j12 (Autodesk Fusion 360 design; units mm, degrees)
part number: 2026-05-31-16-27-39-001
Autodesk Fusion 360 part; units mm, degrees
sketch "Sketch1" plane through (0, 0, 0) normal (0, 0, 1) x (1, 0, 0)
  line L0 (0, 0) -> (50, 0)
  line L1 (50, 0) -> (50, 110)
  line L2 (50, 110) -> (0, 110)
  line L3 (0, 110) -> (0, 0)
  dimension "d1" = 50
  dimension "d2" = 110
  constraint horizontal L0
  constraint vertical L1
  constraint horizontal L2
  constraint vertical L3
  constraint coincident L0.start L3.end
  measures "d1" distance of L0.start L0.end
  measures "d2" distance of L0.start L2.end
extrude "Extrude1" add sketch "Sketch1" along normal blind 5
sketch "Sketch2" plane through (0, 0, 5) normal (0, 0, 1) x (-1, 0, 0)
  line L0 (0, -110) -> (0, 0)
  line L1 (0, 0) -> (-50, 0)
  line L2 (-50, 0) -> (-50, -110)
  line L3 (-50, -110) -> (0, -110)
  circle A0 centre (-5, -5) radius 4
  circle A1 centre (-15, -5) radius 4
  circle A2 centre (-25, -5) radius 4
  circle A3 centre (-35, -5) radius 4
  circle A4 centre (-45, -5) radius 4
  circle A5 centre (-5, -15) radius 4
  circle A6 centre (-15, -15) radius 4
  circle A7 centre (-25, -15) radius 4
  circle A8 centre (-35, -15) radius 4
  circle A9 centre (-45, -15) radius 4
  circle A10 centre (-25, -35) radius 4
  circle A11 centre (-5, -25) radius 4
  circle A12 centre (-35, -35) radius 4
  circle A13 centre (-5, -35) radius 4
  circle A14 centre (-25, -25) radius 4
  circle A15 centre (-15, -25) radius 4
  circle A16 centre (-45, -25) radius 4
  circle A17 centre (-35, -25) radius 4
  circle A18 centre (-45, -35) radius 4
  circle A19 centre (-15, -35) radius 4
  circle A20 centre (-5, -75) radius 4
  circle A21 centre (-25, -65) radius 4
  circle A22 centre (-45, -65) radius 4
  circle A23 centre (-45, -75) radius 4
  circle A24 centre (-5, -65) radius 4
  circle A25 centre (-35, -75) radius 4
  circle A26 centre (-35, -65) radius 4
  circle A27 centre (-25, -75) radius 4
  circle A28 centre (-15, -75) radius 4
  circle A29 centre (-35, -55) radius 4
  circle A30 centre (-15, -65) radius 4
  circle A31 centre (-15, -45) radius 4
  circle A32 centre (-5, -45) radius 4
  circle A33 centre (-25, -55) radius 4
  circle A34 centre (-15, -55) radius 4
  circle A35 centre (-25, -45) radius 4
  circle A36 centre (-45, -45) radius 4
  circle A37 centre (-5, -55) radius 4
  circle A38 centre (-45, -55) radius 4
  circle A39 centre (-35, -45) radius 4
  circle A40 centre (-15, -105) radius 4
  circle A41 centre (-5, -95) radius 4
  circle A42 centre (-45, -105) radius 4
  circle A43 centre (-45, -95) radius 4
  circle A44 centre (-25, -105) radius 4
  circle A45 centre (-15, -95) radius 4
  circle A46 centre (-45, -85) radius 4
  circle A47 centre (-25, -85) radius 4
  circle A48 centre (-35, -85) radius 4
  circle A49 centre (-35, -105) radius 4
  circle A50 centre (-35, -95) radius 4
  circle A51 centre (-25, -95) radius 4
  circle A52 centre (-5, -105) radius 4
  circle A53 centre (-5, -85) radius 4
  circle A54 centre (-15, -85) radius 4
  dimension "d5" = 8
  dimension "d6" = 8
  dimension "d7" = 8
  dimension "d8" = 8
  dimension "d9" = 8
  dimension "d10" = 8
  dimension "d11" = 8
  dimension "d12" = 8
  dimension "d13" = 8
  dimension "d14" = 8
  dimension "d15" = 8
  dimension "d16" = 8
  dimension "d17" = 8
  dimension "d18" = 8
  dimension "d19" = 8
  dimension "d20" = 8
  dimension "d21" = 8
  dimension "d22" = 8
  dimension "d23" = 8
  dimension "d24" = 8
  dimension "d25" = 8
  dimension "d26" = 8
  dimension "d27" = 8
  dimension "d28" = 8
  dimension "d29" = 8
  dimension "d30" = 8
  dimension "d31" = 8
  dimension "d32" = 8
  dimension "d33" = 8
  dimension "d34" = 8
  dimension "d35" = 8
  dimension "d36" = 8
  dimension "d37" = 8
  dimension "d38" = 8
  dimension "d39" = 8
  dimension "d40" = 8
  dimension "d41" = 8
  dimension "d42" = 8
  dimension "d43" = 8
  dimension "d44" = 8
  dimension "d45" = 8
  dimension "d46" = 8
  dimension "d47" = 8
  dimension "d48" = 8
  dimension "d49" = 8
  dimension "d50" = 8
  dimension "d51" = 8
  dimension "d52" = 8
  dimension "d53" = 8
  dimension "d54" = 8
  dimension "d55" = 8
  dimension "d56" = 8
  dimension "d57" = 8
  dimension "d58" = 8
  dimension "d59" = 8
  measures "d5" diameter of A0
  measures "d6" diameter of A1
  measures "d7" diameter of A2
  measures "d8" diameter of A3
  measures "d9" diameter of A4
  measures "d10" diameter of A5
  measures "d11" diameter of A6
  measures "d12" diameter of A7
  measures "d13" diameter of A8
  measures "d14" diameter of A9
  measures "d15" diameter of A11
  measures "d16" diameter of A15
  measures "d17" diameter of A14
  measures "d18" diameter of A17
  measures "d19" diameter of A16
  measures "d20" diameter of A13
  measures "d21" diameter of A19
  measures "d22" diameter of A10
  measures "d23" diameter of A12
  measures "d24" diameter of A18
  measures "d25" diameter of A32
  measures "d26" diameter of A31
  measures "d27" diameter of A35
  measures "d28" diameter of A39
  measures "d29" diameter of A36
  measures "d30" diameter of A37
  measures "d31" diameter of A34
  measures "d32" diameter of A33
  measures "d33" diameter of A29
  measures "d34" diameter of A38
  measures "d35" diameter of A24
  measures "d36" diameter of A30
  measures "d37" diameter of A21
  measures "d38" diameter of A26
  measures "d39" diameter of A22
  measures "d40" diameter of A20
  measures "d41" diameter of A28
  measures "d42" diameter of A27
  measures "d43" diameter of A25
  measures "d44" diameter of A23
  measures "d45" diameter of A53
  measures "d46" diameter of A54
  measures "d47" diameter of A47
  measures "d48" diameter of A48
  measures "d49" diameter of A46
  measures "d50" diameter of A41
  measures "d51" diameter of A45
  measures "d52" diameter of A51
  measures "d53" diameter of A50
  measures "d54" diameter of A43
  measures "d55" diameter of A52
  measures "d56" diameter of A40
  measures "d57" diameter of A44
  measures "d58" diameter of A49
  measures "d59" diameter of A42
extrude "Extrude2" cut sketch "Sketch2" against normal blind 20 contours A0 | A1 | A2 | A3 | A4 | A5 | A6 | A7 | A8 | A9 | A10 | A11 | A12 | A13 | A14 | A15 | A16 | A17 | A18 | A19 | A20 | A21 | A22 | A23 | A24 | A25 | A26 | A27 | A28 | A29 | A30 | A31 | A32 | A33 | A34 | A35 | A36 | A37 | A38 | A39 | A40 | A41 | A42 | A43 | A44 | A45 | A46 | A47 | A48 | A49 | A50 | A51 | A52 | A53 | A54
extrude "Extrude3" add 1 faces at (16.6667, 0, 1.6667) along direction (0, -1, 0) blind 5
sketch "Sketch3" plane through (0, 0, 5) normal (0, 0, 1) x (-1, 0, 0)
  line L0 (0, -110) -> (0, 5)
  line L1 (0, 5) -> (-50, 5)
  line L2 (-50, 5) -> (-50, -110)
  line L3 (-50, -110) -> (0, -110)
  circle A0 centre (-5, -105) radius 4
  circle A1 centre (-45, -105) radius 4
  circle A2 centre (-35, -5) radius 4
  circle A3 centre (-15, -15) radius 4
  circle A4 centre (-45, -25) radius 4
  circle A5 centre (-15, -45) radius 4
  circle A6 centre (-5, -35) radius 4
  circle A7 centre (-25, -95) radius 4
  circle A8 centre (-5, -65) radius 4
  circle A9 centre (-45, -65) radius 4
  circle A10 centre (-25, -65) radius 4
  circle A11 centre (-45, -95) radius 4
  circle A12 centre (-45, -85) radius 4
  circle A13 centre (-5, -85) radius 4
  circle A14 centre (-15, -85) radius 4
  circle A15 centre (-35, -45) radius 4
  circle A16 centre (-35, -75) radius 4
  circle A17 centre (-5, -75) radius 4
  circle A18 centre (-35, -55) radius 4
  circle A19 centre (-25, -75) radius 4
  circle A20 centre (-25, -55) radius 4
  circle A21 centre (-45, -35) radius 4
  circle A22 centre (-5, -25) radius 4
  circle A23 centre (-15, -35) radius 4
  circle A24 centre (-25, -15) radius 4
  circle A25 centre (-45, -5) radius 4
  circle A26 centre (-5, -5) radius 4
  circle A27 centre (-15, -105) radius 4
  circle A28 centre (-35, -105) radius 4
  circle A29 centre (-25, -5) radius 4
  circle A30 centre (-25, -35) radius 4
  circle A31 centre (-35, -15) radius 4
  circle A32 centre (-35, -25) radius 4
  circle A33 centre (-5, -45) radius 4
  circle A34 centre (-35, -95) radius 4
  circle A35 centre (-45, -55) radius 4
  circle A36 centre (-5, -55) radius 4
  circle A37 centre (-15, -65) radius 4
  circle A38 centre (-45, -75) radius 4
  circle A39 centre (-5, -95) radius 4
  circle A40 centre (-45, -45) radius 4
  circle A41 centre (-35, -85) radius 4
  circle A42 centre (-25, -45) radius 4
  circle A43 centre (-15, -95) radius 4
  circle A44 centre (-35, -65) radius 4
  circle A45 centre (-25, -85) radius 4
  circle A46 centre (-15, -75) radius 4
  circle A47 centre (-15, -55) radius 4
  circle A48 centre (-25, -25) radius 4
  circle A49 centre (-35, -35) radius 4
  circle A50 centre (-15, -25) radius 4
  circle A51 centre (-5, -15) radius 4
  circle A52 centre (-45, -15) radius 4
  circle A53 centre (-15, -5) radius 4
  circle A54 centre (-25, -105) radius 4
  line L4 (0, 5) -> (-50, 5)
  line L5 (-50, 5) -> (-50, 0)
  line L6 (-50, 0) -> (0, 0)
  line L7 (0, 0) -> (0, 5)
  constraint horizontal L4
  constraint vertical L5
  constraint horizontal L6
  constraint vertical L7
  constraint coincident L2 L5.end
  constraint coincident L0.end L1.start
extrude "Extrude4" add sketch "Sketch3" along normal blind 42 contours L0 L1 L2 L4 L5 L6 L7
extrude "Extrude5" add 1 faces at (50, 35, 1.6667) along direction (1, 0, 0) blind 5
extrude "Extrude6" add 1 faces at (0, 35, 1.6667) along direction (-1, 0, 0) blind 5
sketch "Sketch4" plane through (0, 0, 0) normal (0, 1, 0) x (-1, 0, 0)
  line L0 (-55, 5) -> (5, 5)
  line L1 (5, 5) -> (5, 47)
  line L2 (5, 47) -> (-55, 47)
  line L3 (-55, 47) -> (-55, 5)
  line L4 (0, 47) -> (5, 47)
  line L5 (5, 47) -> (5, 5)
  line L6 (5, 5) -> (0, 5)
  line L7 (0, 5) -> (0, 47)
  line L8 (-55, 47) -> (-50, 47)
  line L9 (-50, 47) -> (-50, 5)
  line L10 (-50, 5) -> (-55, 5)
  line L11 (-55, 5) -> (-55, 47)
  constraint horizontal L4
  constraint vertical L5
  constraint horizontal L6
  constraint vertical L7
  constraint coincident L0.end L1.start
  constraint horizontal L8
  constraint vertical L9
  constraint horizontal L10
  constraint vertical L11
  constraint coincident L0 L9.end
  constraint coincident L2.end L3.start
extrude "Extrude7" add sketch "Sketch4" along normal blind 110 contours L0 L2 L3 L8 L9 L10 L11 | L0 L1 L2 L4 L5 L6 L7
sketch "Sketch5" plane through (-5, 0, 0) normal (-1, 0, 0) x (0, -1, 0)
  line L0 (-110, 0) -> (5, 0)
  line L1 (5, 0) -> (5, 47)
  line L2 (5, 47) -> (-110, 47)
  line L3 (-110, 47) -> (-110, 0)
  circle A0 centre (-105, 10) radius 4
  circle A1 centre (-95, 10) radius 4
  circle A2 centre (-85, 10) radius 4
  circle A3 centre (-75, 10) radius 4
  circle A4 centre (-65, 10) radius 4
  circle A5 centre (-55, 10) radius 4
  circle A6 centre (-45, 10) radius 4
  circle A7 centre (-35, 10) radius 4
  circle A8 centre (-25, 10) radius 4
  circle A9 centre (-15, 10) radius 4
  circle A10 centre (-6, 10) radius 4
  circle A11 centre (-25, 20) radius 4
  circle A12 centre (-75, 20) radius 4
  circle A13 centre (-35, 20) radius 4
  circle A14 centre (-85, 20) radius 4
  circle A15 centre (-105, 20) radius 4
  circle A16 centre (-6, 20) radius 4
  circle A17 centre (-15, 20) radius 4
  circle A18 centre (-65, 20) radius 4
  circle A19 centre (-45, 20) radius 4
  circle A20 centre (-55, 20) radius 4
  circle A21 centre (-95, 20) radius 4
  circle A22 centre (-6, 40) radius 4
  circle A23 centre (-15, 40) radius 4
  circle A24 centre (-25, 40) radius 4
  circle A25 centre (-75, 40) radius 4
  circle A26 centre (-85, 40) radius 4
  circle A27 centre (-65, 30) radius 4
  circle A28 centre (-95, 30) radius 4
  circle A29 centre (-35, 40) radius 4
  circle A30 centre (-35, 30) radius 4
  circle A31 centre (-15, 30) radius 4
  circle A32 centre (-25, 30) radius 4
  circle A33 centre (-6, 30) radius 4
  circle A34 centre (-45, 40) radius 4
  circle A35 centre (-95, 40) radius 4
  circle A36 centre (-105, 40) radius 4
  circle A37 centre (-65, 40) radius 4
  circle A38 centre (-55, 40) radius 4
  circle A39 centre (-45, 30) radius 4
  circle A40 centre (-75, 30) radius 4
  circle A41 centre (-105, 30) radius 4
  circle A42 centre (-85, 30) radius 4
  circle A43 centre (-55, 30) radius 4
  dimension "d72" = 8
  dimension "d73" = 8
  dimension "d74" = 8
  dimension "d75" = 8
  dimension "d76" = 8
  dimension "d77" = 8
  dimension "d78" = 8
  dimension "d79" = 8
  dimension "d80" = 8
  dimension "d81" = 8
  dimension "d82" = 8
  dimension "d83" = 8
  dimension "d84" = 8
  dimension "d85" = 8
  dimension "d86" = 8
  dimension "d87" = 8
  dimension "d88" = 8
  dimension "d89" = 8
  dimension "d90" = 8
  dimension "d91" = 8
  dimension "d92" = 8
  dimension "d93" = 8
  dimension "d94" = 8
  dimension "d95" = 8
  dimension "d96" = 8
  dimension "d97" = 8
  dimension "d98" = 8
  dimension "d99" = 8
  dimension "d100" = 8
  dimension "d101" = 8
  dimension "d102" = 8
  dimension "d103" = 8
  dimension "d104" = 8
  dimension "d105" = 8
  dimension "d106" = 8
  dimension "d107" = 8
  dimension "d108" = 8
  dimension "d109" = 8
  dimension "d110" = 8
  dimension "d111" = 8
  dimension "d112" = 8
  dimension "d113" = 8
  dimension "d114" = 8
  dimension "d115" = 8
  measures "d72" diameter of A0
  measures "d73" diameter of A1
  measures "d74" diameter of A2
  measures "d75" diameter of A3
  measures "d76" diameter of A4
  measures "d77" diameter of A5
  measures "d78" diameter of A6
  measures "d79" diameter of A7
  measures "d80" diameter of A8
  measures "d81" diameter of A9
  measures "d82" diameter of A10
  measures "d83" diameter of A15
  measures "d84" diameter of A21
  measures "d85" diameter of A14
  measures "d86" diameter of A12
  measures "d87" diameter of A18
  measures "d88" diameter of A20
  measures "d89" diameter of A19
  measures "d90" diameter of A13
  measures "d91" diameter of A11
  measures "d92" diameter of A17
  measures "d93" diameter of A16
  measures "d94" diameter of A41
  measures "d95" diameter of A28
  measures "d96" diameter of A42
  measures "d97" diameter of A40
  measures "d98" diameter of A27
  measures "d99" diameter of A43
  measures "d100" diameter of A39
  measures "d101" diameter of A30
  measures "d102" diameter of A32
  measures "d103" diameter of A31
  measures "d104" diameter of A33
  measures "d105" diameter of A36
  measures "d106" diameter of A35
  measures "d107" diameter of A26
  measures "d108" diameter of A25
  measures "d109" diameter of A37
  measures "d110" diameter of A38
  measures "d111" diameter of A34
  measures "d112" diameter of A29
  measures "d113" diameter of A24
  measures "d114" diameter of A23
  measures "d115" diameter of A22
extrude "Extrude8" cut sketch "Sketch5" against normal blind 80 contours A0 | A1 | A2 | A3 | A4 | A5 | A6 | A7 | A8 | A9 | A10 | A11 | A12 | A13 | A14 | A15 | A16 | A17 | A18 | A19 | A20 | A21 | A22 | A23 | A24 | A25 | A26 | A27 | A28 | A29 | A30 | A31 | A32 | A33 | A34 | A35 | A36 | A37 | A38 | A39 | A40 | A41 | A42 | A43
sketch "Sketch6" plane through (0, -5, 0) normal (0, -1, 0) x (1, 0, 0)
  line L0 (-5, 0) -> (55, 0)
  line L1 (55, 0) -> (55, 47)
  line L2 (55, 47) -> (-5, 47)
  line L3 (-5, 47) -> (-5, 0)
  line L4 (-2, 44) -> (52, 44)
  line L5 (52, 44) -> (52, 8)
  line L6 (52, 8) -> (-2, 8)
  line L7 (-2, 8) -> (-2, 44)
  constraint horizontal L4
  constraint vertical L5
  constraint horizontal L6
  constraint vertical L7
extrude "Extrude9" cut sketch "Sketch6" against normal blind 2 contours L4 L5 L6 L7
sketch "Sketch7" plane through (0, -3, 0) normal (0, -1, 0) x (1, 0, 0)
  line L0 (-2, 8) -> (52, 8)
  line L1 (52, 8) -> (52, 44)
  line L2 (52, 44) -> (-2, 44)
  line L3 (-2, 44) -> (-2, 8)
  circle A0 centre (25, 26) radius 18.5
  line L4 (25, 44.5) -> (25, 34.5)
  line L5 (25, 7.5) -> (25, 17.5)
  circle A1 centre (25, 17.5) radius 1.45
  circle A2 centre (25, 34.5) radius 1.45
  dimension "d120" = 37
  dimension "d121" = 10
  dimension "d122" = 10
  dimension "d123" = 2.9
  dimension "d124" = 2.9
  constraint coincident A0 L4.start
  constraint perpendicular L2 L4
  constraint coincident A0 L5.start
  constraint perpendicular L0 L5
  constraint coincident L5.end A1.centre
  constraint coincident L4.end A2.centre
  measures "d120" diameter of A0
  measures "d121" distance of L4.start L4.end
  measures "d122" distance of L5.start L5.end
  measures "d123" diameter of A1
  measures "d124" diameter of A2
extrude "Extrude10" cut sketch "Sketch7" against normal blind 6 contours A1 | A2
extrude "Extrude11" add 1 faces at (-3.3333, 35, 47) along direction (0, 0, 1) blind 5
sketch "Sketch8" plane through (0, 0, 0) normal (0, 1, 0) x (-1, 0, 0)
  circle A0 centre (-25, 17.5) radius 1.45
  circle A1 centre (-25, 34.5) radius 1.45
  line L0 (0, 5) -> (0, 52)
  line L1 (0, 52) -> (-50, 52)
  line L2 (-50, 52) -> (-50, 5)
  line L3 (-50, 5) -> (0, 5)
  line L4 (-55, 52) -> (5, 52)
  line L5 (5, 52) -> (5, 47)
  line L6 (5, 47) -> (-55, 47)
  line L7 (-55, 47) -> (-55, 52)
  constraint horizontal L4
  constraint vertical L5
  constraint horizontal L6
  constraint vertical L7
extrude "Extrude12" add sketch "Sketch8" along normal blind 45 contours L0 L1 L2 L4 L6
sketch "Sketch9" plane through (0, 0, 52) normal (0, 0, 1) x (-1, 0, 0)
  line L0 (5, 5) -> (-55, 5)
  line L1 (-55, 5) -> (-55, -110)
  line L2 (-55, -110) -> (-50, -110)
  line L3 (-50, -110) -> (-50, -45)
  line L4 (-50, -45) -> (0, -45)
  line L5 (0, -45) -> (0, -110)
  line L6 (0, -110) -> (5, -110)
  line L7 (5, -110) -> (5, 5)
  circle A0 centre (-25, -20) radius 19.1257
extrude "Extrude13" cut sketch "Sketch9" against normal blind 15 contours A0
sketch "Sketch10" plane through (0, 0, 52) normal (0, 0, 1) x (-1, 0, 0)
  circle A0 centre (-25, -20) radius 19.1257
  line L0 (5, 5) -> (-55, 5)
  line L1 (-55, 5) -> (-55, -110)
  line L2 (-55, -110) -> (-50, -110)
  line L3 (-50, -110) -> (-50, -45)
  line L4 (-50, -45) -> (0, -45)
  line L5 (0, -45) -> (0, -110)
  line L6 (0, -110) -> (5, -110)
  line L7 (5, -110) -> (5, 5)
  circle A1 centre (-25, -20) radius 22.4722
  circle A2 centre (-25, -20) radius 19.1257
  constraint concentric A0 A1
  constraint concentric A1 A2
extrude "Extrude14" add sketch "Sketch10" along normal blind 40 contours A1
sketch "Sketch11" plane through (0, -5, 0) normal (0, -1, 0) x (1, 0, 0)
  line L0 (52, 44) -> (52, 8)
  line L1 (52, 8) -> (-2, 8)
  line L2 (-2, 8) -> (-2, 44)
  line L3 (-2, 44) -> (52, 44)
  line L4 (-5, 0) -> (55, 0)
  line L5 (55, 0) -> (55, 52)
  line L6 (55, 52) -> (-5, 52)
  line L7 (-5, 52) -> (-5, 0)
  circle A0 centre (12, 85) radius 1.25
  circle A1 centre (38, 85) radius 1.25
  circle A2 centre (13, 59) radius 1.25
  circle A3 centre (40, 59) radius 1.25
  dimension "d135" = 2.5
  dimension "d136" = 2.5
  dimension "d137" = 2.5
  dimension "d138" = 2.5
  measures "d135" diameter of A0
  measures "d136" diameter of A1
  measures "d137" diameter of A2
  measures "d138" diameter of A3
extrude "Extrude15" cut sketch "Sketch11" against normal blind 56 contours A0 | A1 | A2 | A3
fillet "Fillet1" radius 3 1 edges at (25, -5, 52)
fillet "Fillet2" radius 0.75 1 edges at (23.6481, -3, 35.0243)
fillet "Fillet3" radius 0.75 1 edges at (23.6481, -3, 18.0243)
